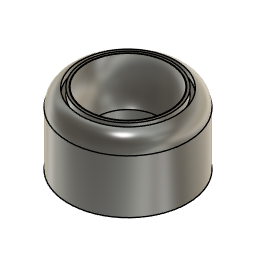
Air Vents V3 (Autodesk Fusion 360 design; units mm, degrees)
Autodesk Fusion 360 part; units mm, degrees
sketch "Sketch1" plane through (0, 0, 0) normal (0, 0, 1) x (1, 0, 0)
  circle A0 centre (-2.9518, -4.3204) radius 23.5
  circle A1 centre (-2.9518, -4.3204) radius 16
  circle A2 centre (-2.9518, -4.3204) radius 13.5
  circle A3 centre (-2.9518, -4.3204) radius 12.5
  circle A4 centre (-2.9518, -4.3204) radius 11.5
  circle A5 centre (-2.9518, -4.3204) radius 20
  dimension "d1" = 47
  dimension "d2" = 32
  dimension "d3" = 27
  dimension "d4" = 25
  dimension "d5" = 23
  dimension "d112" = 40
  constraint concentric A0 A1
  constraint concentric A1 A2
  constraint concentric A1 A3
  constraint concentric A0 A4
  constraint concentric A3 A5
  measures "d1" diameter of A0
  measures "d2" diameter of A1
  measures "d3" diameter of A2
  measures "d4" diameter of A3
  measures "d5" diameter of A4
  measures "d112" diameter of A5
extrude "Extrude1" add sketch "Sketch1" along normal blind 11 contours A5 makes body 1
extrude "Extrude2" add sketch "Sketch1" along normal blind 9 and the other way blind -11 contours A0 bodies 1
copy_body "Body->Comp1" bodies 1 removing the originals makes body 2 in component "External Case"
extrude "Extrude3" add sketch "Sketch1" along normal blind 26 separate body contours A2 makes body 3
extrude "Extrude4" add sketch "Sketch1" along normal blind 31 contours A3 bodies 3
extrude "Extrude1'" add 1 faces at (15.5808, -6.1089, 0) along direction (0, 0, -1) blind 11 on bodies 2 bodies 2 in component "External Case"
extrude "Extrude5" add 1 faces at (9.8313, -4.9911, 0) along direction (0, 0, -1) blind 10 on bodies 3 bodies 3
copy_body "Body->Comp2" bodies 3 removing the originals makes body 4 in component "Internal Case"
sketch "Sketch1 (2)" plane through (0, 0, 31) normal (0, 0, 1) x (-1, 0, 0) in component "Internal block"
  circle A0 centre (2.9518, 4.3204) radius 11.5
  circle A1 centre (2.9518, 4.3204) radius 2.5
  circle A2 centre (2.9518, 4.3204) radius 12.5
  circle A3 centre (2.9518, 4.3204) radius 11.25
  dimension "d22" = 5
  dimension "d201" = 22.5
  measures "d22" diameter of A1
  measures "d201" diameter of A3
extrude "Extrude1''" add sketch "Sketch1 (2)" against normal blind 2 separate body contours A1 | A3 makes body 5 in component "Internal block"
extrude "Extrude2'" add sketch "Sketch1 (2)" along normal blind 3 contours A1 bodies 5 in component "Internal block"
fillet "Fillet1" radius 0.75 tangency weight 0.47649 1 edges at (-0.621, -3.4164, 34) on bodies 5 in component "Internal block"
move_body "Move1" bodies 5 to x (1, 0, 0) y (0, 1, 0) z (0, 0, 1) at (0, 0, -20) in component "Internal block"
sphere "SpherePrimitive1" add diameter 35 placed x (1, 0, 0) y (0, -1, 0) z (0, 0, -1) at (-2.9518, -4.3204, -10) separate body makes body 6 in component "Internal Case"
move_body "Move1'" bodies 6 to x (1, 0, 0) y (0, 1, 0) z (0, 0, 1) at (0, 0, -7) in component "Internal Case"
sphere "SpherePrimitive1'" add diameter 39 placed x (1, 0, 0) y (0, -1, 0) z (0, 0, -1) at (-2.9518, -4.3204, -11) separate body makes body 7
split "Split2" by plane through (0, 0, -10) normal (0, 0, -1) bodies 6 makes body 8 at (10.2147, -6.642, -5.7083) in component "Internal Case"
combine "Combine2" operation add target body 4 tool bodies 8 6 in component "Internal Case"
move_body "Move2" bodies 7 to x (1, 0, 0) y (0, 1, 0) z (0, 0, 1) at (0, 0, -9.5)
ref_plane "WorkPlane2" through (0, 0, -12) normal (0, 0, 1) x (1, 0, 0)
split "Split1" by plane through (0, 0, -12) normal (0, 0, 1) bodies 7 makes body 9 at (11.3458, -6.8415, -7.4819)
delete_body "RemoveBody6" bodies 9
ref_plane "WorkPlane3" through (0, 0, 0) normal (1, 0, 0) x (0, 1, 0)
ref_plane "WorkPlane4" through (0, 0, -45) normal (0, 0, 1) x (1, 0, 0)
sketch "Sketch10" plane through (0, 0, -45) normal (0, 0, 1) x (1, 0, 0)
  line L0 (19.5471, 18.1746) -> (-25.4529, 18.1746)
  line L1 (-25.4529, 18.1746) -> (-25.4529, -26.8254)
  line L2 (-25.4529, -26.8254) -> (19.5471, -26.8254)
  line L3 (19.5471, -26.8254) -> (19.5471, 18.1746)
  line L4 (19.5471, 18.1746) -> (-25.4529, -26.8254) construction
  line L5 (-25.4529, 18.1746) -> (19.5471, -26.8254) construction
  point P0 (-2.9529, -4.3254)
  dimension "d50" = 45
  dimension "d51" = 45
  constraint horizontal L0
  constraint perpendicular L0 L1
  constraint parallel L0 L2
  constraint parallel L1 L3
  constraint coincident L4 P0
  constraint coincident L5 P0
  measures "d50" distance of L1.end L2.end
  measures "d51" distance of L0.end L1.end
sketch "Sketch12" plane through (0, 0, -12) normal (0, 0, 1) x (-1, 0, 0)
  circle A0 centre (2.9518, 4.3204) radius 17.5499
  line L0 (-19.5482, 26.8204) -> (25.4518, 26.8204)
  line L1 (25.4518, 26.8204) -> (25.4518, -18.1796)
  line L2 (25.4518, -18.1796) -> (-19.5482, -18.1796)
  line L3 (-19.5482, -18.1796) -> (-19.5482, 26.8204)
  line L4 (-19.5482, 26.8204) -> (25.4518, -18.1796) construction
  line L5 (25.4518, 26.8204) -> (-19.5482, -18.1796) construction
  line L6 (27.9518, -20.6796) -> (-22.0482, -20.6796)
  line L7 (-22.0482, -20.6796) -> (-22.0482, 29.3204)
  line L8 (-22.0482, 29.3204) -> (27.9518, 29.3204)
  line L9 (27.9518, 29.3204) -> (27.9518, -20.6796)
  line L10 (27.9518, -20.6796) -> (-22.0482, 29.3204) construction
  line L11 (-22.0482, -20.6796) -> (27.9518, 29.3204) construction
  point P0 (2.9518, 4.3204)
  point P1 (2.9518, 4.3204)
  dimension "d57" = 45
  dimension "d58" = 45
  dimension "d113" = 50
  dimension "d114" = 50
  constraint horizontal L0
  constraint perpendicular L0 L1
  constraint parallel L0 L2
  constraint parallel L1 L3
  constraint coincident L4 P1
  constraint coincident L5 P1
  constraint coincident P0 A0.centre
  constraint horizontal L6
  constraint perpendicular L6 L7
  constraint parallel L6 L8
  constraint parallel L7 L9
  constraint coincident L10 P1
  constraint coincident L11 P1
  constraint coincident P1 P0
  measures "d57" distance of L1.end L2.end
  measures "d58" distance of L0.end L1.end
  measures "d113" distance of L7.end L8.end
  measures "d114" distance of L6.end L7.end
extrude "Extrude8" add sketch "Sketch12" against normal blind 30 contours A0 | L0 L1 L2 L3 | L6 L7 L8 L9 bodies 7
combine "Combine1" operation cut target body 7 tool bodies 4 keep tools
move_face "OffsetFaces1" offset -0.5 1 faces at (10.0519, -16.029, -16.753) on bodies 7
fillet "Fillet1'" radius 25 4 edges at (-27.9518, -29.3204, -27) (22.0482, -29.3204, -27) (-27.9518, 20.6796, -27) (22.0482, 20.6796, -27) on bodies 7
fillet "Fillet2" radius 7.5 1 edges at (7.137, -27.1943, -12) on bodies 7
sketch "Sketch22" plane through (0, 0, 31) normal (0, 0, 1) x (-1, 0, 0)
  circle A0 centre (2.9518, 4.3204) radius 11.5
  circle A1 centre (2.9518, 4.3204) radius 12.5
  circle A2 centre (2.9518, 4.3204) radius 12.5
  dimension "d173" = 25
  measures "d173" diameter of A2
extrude "Extrude22" cut sketch "Sketch22" against normal blind 89 contours A0 bodies 7
extrude "Extrude2''" cut sketch "Sketch22" against normal blind 89 contours A0 bodies 4 in component "Internal Case"
sketch "Sketch23" plane through (0, 0, -42) normal (0, 0, -1) x (1, 0, 0)
  circle A0 centre (-2.9518, 4.3204) radius 11.5
  circle A1 centre (-2.9518, 4.3204) radius 25
  circle A2 centre (-2.9518, 4.3204) radius 13
  dimension "d148" = 26
  constraint concentric A0 A2
  measures "d148" diameter of A2
extrude "Extrude23" cut sketch "Sketch23" against normal blind 13 contours A2 bodies 7
sketch "Sketch27" plane through (0, 0, -4) normal (0, 0, -1) x (1, 0, 0)
  circle A0 centre (-2.9518, 4.3204) radius 20
  circle A1 centre (-2.9518, 4.3204) radius 16
  circle A2 centre (-2.9518, 4.3204) radius 18.5
  dimension "d165" = 37
  constraint concentric A0 A2
  measures "d165" diameter of A2
extrude "Extrude25" cut sketch "Sketch27" along normal blind 11 contours A0 bodies 7
extrude "Extrude27" add sketch "Sketch27" along normal blind 11 separate body contours A0 makes body 10
copy_body "CutPasteBodies4" bodies 10 body 10 seen with x (1, 0, 0) y (0, 1, 0) z (0, 0, 1) at (0, 0, -7) removing the originals makes body 11 in component "External Case"
move_face "OffsetFaces3" offset -0.05 1 faces at (-14.2004, 12.2165, -14.1427) on bodies 7
sketch "Sketch28" plane through (0, 0, -42) normal (0, 0, -1) x (1, 0, 0)
  circle A0 centre (-2.9518, 4.3204) radius 13
  circle A1 centre (-2.9518, 4.3204) radius 25
  circle A2 centre (-2.9518, 4.3204) radius 13
  circle A3 centre (-2.9518, 4.3204) radius 15
  circle A4 centre (-2.9518, 4.3204) radius 20
  dimension "d174" = 30
  dimension "d175" = 40
  constraint concentric A0 A2
  constraint concentric A2 A3
  constraint concentric A3 A4
  measures "d174" diameter of A3
  measures "d175" diameter of A4
extrude "Extrude28" cut sketch "Sketch28" against normal blind 5 contours A4 bodies 7
extrude "Extrude29" add 1 faces at (15.2512, -2.5816, -37) along direction (0, 0, -1) blind 20 separate body on bodies 7 makes body 12
copy_body "Body->Comp3" bodies 12 removing the originals makes body 13 in component "Hose Connector"
move_face "OffsetFaces4" offset -0.05 1 faces at (-22.927, -3.3235, -40.3333) on bodies 7
sketch "Sketch3" plane through (0, 0, 14) normal (0, 0, 1) x (-1, 0, 0) in component "Internal block"
  spline S0 degree 3 poles (1.2018, 4.3204) (1.2018, 4.8935) (1.5039, 5.4581) (2.3791, 6.0421) (2.8897, 6.1337) (3.8161, 5.9139) (4.2267, 5.6092) (4.6944, 4.8051) (4.7606, 4.3178) (4.5378, 3.47) (4.2798, 3.106) (3.6128, 2.6548) (3.2203, 2.5486) (2.4602, 2.5993) (2.0946, 2.7491) (1.5759, 3.1958) (1.3969, 3.4603) (1.234, 3.9346) (1.2018, 4.1275) (1.2018, 4.3204) knots -1.094554 -1.094554 -1.094554 -1.094554 -0.923405 -0.923405 -0.780335 -0.780335 -0.63905 -0.63905 -0.502512 -0.502512 -0.377257 -0.377257 -0.262027 -0.262027 -0.149781 -0.149781 -0.057608 -0.057608 0 0 0 0
  line L0 (1.2018, 4.3204) -> (4.7018, 4.3204)
  line L1 (5.8592, 4.8204) -> (0.0444, 4.8204)
  line L2 (0.0444, 4.8204) -> (0.0444, 3.8204)
  line L3 (0.0444, 3.8204) -> (5.8592, 3.8204)
  line L4 (5.8592, 3.8204) -> (5.8592, 4.8204)
  line L5 (5.8592, 4.8204) -> (0.0444, 3.8204) construction
  line L6 (0.0444, 4.8204) -> (5.8592, 3.8204) construction
  point P0 (2.9518, 4.3204)
  dimension "d181" = 1
  constraint coincident S0.start S0.end
  constraint coincident S0 L0.end
  constraint horizontal L0
  constraint horizontal L1
  constraint perpendicular L1 L2
  constraint parallel L1 L3
  constraint parallel L2 L4
  constraint coincident L5 P0
  constraint coincident L6 P0
  constraint midpoint L0 P0
  measures "d181" distance of L1.end L2.end
extrude "Extrude3'" add sketch "Sketch3" along normal blind 1.5 contours S0 L0 L3 | S0 L0 L1 bodies 5 in component "Internal block"
fillet "Fillet2'" radius 0.5 tangency weight 0.1 6 edges at (-2.9518, -3.8204, 15.5) (-2.9518, -4.8204, 15.5) (-1.2208, -4.5728, 15.5) (-1.2202, -4.0678, 15.5) (-4.6832, -4.0677, 15.5) (-4.6824, -4.5729, 15.5) on bodies 5 in component "Internal block"
fillet "Fillet3" radius 0.84 2 edges at (-2.9518, -3.8204, 14) (-2.9518, -4.8204, 14) on bodies 5 in component "Internal block"
extrude "Extrude4'" add 1 faces at (-4.5266, -8.3329, 9) along direction (0, 0, -1) blind 2 on bodies 5 bodies 5 in component "Internal block"
fillet "Fillet4" radius 2.5 1 edges at (-0.621, -5.2245, 11) on bodies 5 in component "Internal block"
sketch "Sketch30" plane through (0, 0, 0) normal (1, 0, 0) x (0, 1, 0)
  line L0 (-15.5, 11) -> (6.9, 11)
  line L1 (-4.3, 11) -> (-4.3, 9)
  circle A0 centre (-4.3, 9) radius 1.1
  dimension "d202" = 22.4
  dimension "d203" = 2
  dimension "d204" = 2.2
  constraint horizontal L0
  constraint midpoint L0 L1.start
  constraint perpendicular L0 L1
  constraint coincident L1.end A0.centre
  measures "d202" distance of L0.start L0.end
  measures "d203" distance of L1.start L1.end
  measures "d204" diameter of A0
extrude "Extrude6" cut sketch "Sketch30" along normal blind -28 and the other way blind -15 bodies 5 in component "Internal block"
extrude "Extrude4''" cut sketch "Sketch30" along normal blind -28 and the other way blind -15 bodies 4 in component "Internal Case"
ref_plane "WorkPlane7" through (-2.9518, -4.3204, -2) normal (0, 0, -1) x (-1, 0, 0)
split "Split1'" by plane through (-2.9518, -4.3204, -9) normal (0, 0, -1) bodies 2 makes body 14 at (15.5808, -6.1089, -11) in component "External Case"
sketch "Sketch31" plane through (0, 0, -9) normal (0, 0, 1) x (-1, 0, 0) in component "External Case"
  circle A0 centre (2.9518, 4.3204) radius 20
  circle A1 centre (2.9518, 4.3204) radius 16
  circle A2 centre (2.9518, 4.3204) radius 20
  circle A3 centre (2.9518, 4.3204) radius 30
  dimension "d214" = 60
  constraint concentric A0 A2
  constraint concentric A2 A3
  measures "d214" diameter of A3
extrude "Extrude5'" add sketch "Sketch31" against normal blind 3 separate body contours A3 makes body 15 in component "External Case"
copy_body "CutPasteBodies1" bodies 11 15 14 removing the originals makes body 16 makes body 17 makes body 18 in component "Connector"
sketch "Sketch1 (3)" plane through (0, 0, -9) normal (0, 0, -1) x (1, 0, 0) in component "External Case"
  circle A0 centre (-2.9518, 4.3204) radius 16
  circle A1 centre (-2.9518, 4.3204) radius 20
  circle A2 centre (-2.9518, 4.3204) radius 20
  circle A3 centre (-2.9518, 4.3204) radius 16
  line L0 (-2.9518, 20.3204) -> (-2.9518, 24.3204)
  line L1 (-1.4518, 20.8204) -> (-4.4518, 20.8204)
  line L2 (-4.4518, 20.8204) -> (-4.4518, 23.8204)
  line L3 (-4.4518, 23.8204) -> (-1.4518, 23.8204)
  line L4 (-1.4518, 23.8204) -> (-1.4518, 20.8204)
  line L5 (-1.4518, 20.8204) -> (-4.4518, 23.8204) construction
  line L6 (-4.4518, 20.8204) -> (-1.4518, 23.8204) construction
  line L7 (-2.9518, 4.3204) -> (-2.9518, -11.6796)
  line L8 (-2.9518, -11.6796) -> (-2.9518, -15.6796)
  line L9 (-1.4518, -15.1796) -> (-4.4518, -15.1796)
  line L10 (-4.4518, -15.1796) -> (-4.4518, -12.1796)
  line L11 (-4.4518, -12.1796) -> (-1.4518, -12.1796)
  line L12 (-1.4518, -12.1796) -> (-1.4518, -15.1796)
  line L13 (-1.4518, -15.1796) -> (-4.4518, -12.1796) construction
  line L14 (-4.4518, -15.1796) -> (-1.4518, -12.1796) construction
  line L15 (-2.9518, 4.3204) -> (-18.9518, 4.3204)
  line L16 (-18.9518, 4.3204) -> (-22.9518, 4.3204)
  line L17 (-2.9518, 4.3204) -> (13.0482, 4.3204)
  line L18 (13.0482, 4.3204) -> (17.0482, 4.3204)
  line L19 (16.5482, 2.8204) -> (13.5482, 2.8204)
  line L20 (13.5482, 2.8204) -> (13.5482, 5.8204)
  line L21 (13.5482, 5.8204) -> (16.5482, 5.8204)
  line L22 (16.5482, 5.8204) -> (16.5482, 2.8204)
  line L23 (16.5482, 2.8204) -> (13.5482, 5.8204) construction
  line L24 (13.5482, 2.8204) -> (16.5482, 5.8204) construction
  line L25 (-19.4518, 2.8204) -> (-22.4518, 2.8204)
  line L26 (-22.4518, 2.8204) -> (-22.4518, 5.8204)
  line L27 (-22.4518, 5.8204) -> (-19.4518, 5.8204)
  line L28 (-19.4518, 5.8204) -> (-19.4518, 2.8204)
  line L29 (-19.4518, 2.8204) -> (-22.4518, 5.8204) construction
  line L30 (-22.4518, 2.8204) -> (-19.4518, 5.8204) construction
  point P0 (-2.9518, 22.3204)
  point P1 (-2.9518, -13.6796)
  point P2 (15.0482, 4.3204)
  point P3 (-20.9518, 4.3204)
  dimension "d217" = 3
  dimension "d218" = 3
  dimension "d219" = 3
  dimension "d220" = 3
  dimension "d221" = 4
  dimension "d222" = 4
  dimension "d223" = 3
  dimension "d224" = 3
  dimension "d225" = 3
  dimension "d226" = 3
  constraint concentric A0 A2
  constraint concentric A2 A3
  constraint coincident A3 L0.start
  constraint coincident A2 L0.end
  constraint vertical L0
  constraint horizontal L1
  constraint perpendicular L1 L2
  constraint parallel L1 L3
  constraint parallel L2 L4
  constraint coincident L5 P0
  constraint coincident L6 P0
  constraint midpoint L0 P0
  constraint coincident A0.centre A1.centre
  constraint coincident A3 L7.end
  constraint vertical L7
  constraint coincident A2 L8.end
  constraint parallel L7 L8
  constraint horizontal L9
  constraint perpendicular L9 L10
  constraint parallel L9 L11
  constraint parallel L10 L12
  constraint coincident L13 P1
  constraint coincident L14 P1
  constraint midpoint L8 P1
  constraint coincident A3 L15.end
  constraint perpendicular L7 L15
  constraint parallel L15 L16
  constraint coincident A3 L17.end
  constraint perpendicular L7 L17
  constraint parallel L17 L18
  constraint horizontal L19
  constraint perpendicular L19 L20
  constraint parallel L19 L21
  constraint parallel L20 L22
  constraint coincident L23 P2
  constraint coincident L24 P2
  constraint midpoint L18 P2
  constraint horizontal L25
  constraint perpendicular L25 L26
  constraint parallel L25 L27
  constraint parallel L26 L28
  constraint coincident L29 P3
  constraint coincident L30 P3
  constraint midpoint L16 P3
  measures "d217" distance of L2.end L3.end
  measures "d218" distance of L1.end L2.end
  measures "d219" distance of L10.end L11.end
  measures "d220" distance of L9.end L10.end
  measures "d221" distance of L15.end L16.end
  measures "d222" distance of L17.end L18.end
  measures "d223" distance of L20.end L21.end
  measures "d224" distance of L19.end L20.end
  measures "d225" distance of L26.end L27.end
  measures "d226" distance of L25.end L26.end
extrude "Extrude1'''" cut sketch "Sketch1 (3)" along normal blind 1.5 contours L18 L20 L21 L22 | L18 L19 L20 L22 | L0 L1 L2 L3 | L0 L1 L3 L4 | L8 L9 L11 L12 | L8 L9 L10 L11 | L16 L25 L26 L28 | L16 L26 L27 L28 bodies 18 in component "Connector"
move_face "OffsetFaces1'" offset -0.05 16 faces at (-2.4518, 15.1796, -9.5) (-4.4518, 14.1796, -9.5) (-3.4518, 12.1796, -9.5) (-1.4518, 13.1796, -9.5) (13.5482, -3.8204, -9.5) (14.5482, -5.8204, -9.5) (16.5482, -4.8204, -9.5) (15.5482, -2.8204, -9.5) (-3.4518, -23.8204, -9.5) (-1.4518, -22.8204, -9.5) (-2.4518, -20.8204, -9.5) (-4.4518, -21.8204, -9.5) (-20.4518, -2.8204, -9.5) (-19.4518, -4.8204, -9.5) (-21.4518, -5.8204, -9.5) (-22.4518, -3.8204, -9.5) on bodies 18 in component "Connector"
extrude "Extrude6'" add sketch "Sketch1 (3)" along normal blind 1.5 contours L18 L20 L21 L22 | L18 L19 L20 L22 | L0 L1 L2 L3 | L0 L1 L3 L4 | L8 L9 L11 L12 | L8 L9 L10 L11 | L16 L25 L26 L28 | L16 L26 L27 L28 bodies 2 in component "External Case"
component "External Case" placed x (1, 0, 0) y (0, 1, 0) z (0, 0, 1) at (0, 0, 7)
component "Internal block" placed x (1, 0, 0) y (0, 1, 0) z (0, 0, 1) at (0, 0, 0)
component "Internal Case" placed x (1, 0, 0) y (0, 1, 0) z (0, 0, 1) at (0, 0, 0)
component "Hose Connector" placed x (1, 0, 0) y (0, 1, 0) z (0, 0, 1) at (0, 0, 0)
component "Connector" placed x (1, 0, 0) y (0, 1, 0) z (0, 0, 1) at (0, 0, 0) in component "External Case"
named bodies: "Top Half", "Internal Body", "Shell Left", "Connector", "Connector Top", "Connector Ext Ring"
